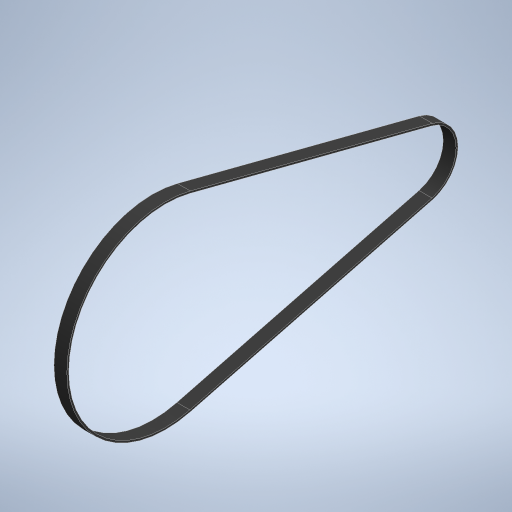
# Autodesk Inventor part: 射出_type1
Saved by Autodesk Inventor 2023 (Build 270158000, 158)
## iProperties
Created: 2022-04-20
Part Number: 射出_type1
Material: ゴム
Document SubType Name: Modeling
Designer: yuta
Density: 0.93 g/cm^3
Appearance: ゴム - 黒
Author: yuta
Autodesk Inventor part; units mm, degrees
ref_plane "YZ Plane" through (0, 0, 0) normal (1, 0, 0) x (0, 1, 0)
ref_plane "XZ Plane" through (0, 0, 0) normal (0, 1, 0) x (-1, 0, 0)
ref_plane "XY Plane" through (0, 0, 0) normal (0, 0, 1) x (1, 0, 0)
sketch "スケッチ1" plane through (0, 0, 0) normal (1, 0, 0) x (0, 1, 0)
  arc A0 (74.0708, -19.125) -> (-74.0708, -19.125) centre (0, 0) ccw
  arc A1 (-25.6585, -206.625) -> (25.6585, -206.625) centre (0, -200) ccw
  line L0 (74.0708, -19.125) -> (25.6585, -206.625)
  line L1 (-74.0708, -19.125) -> (-25.6585, -206.625)
  arc A2 (72.6184, -18.75) -> (-72.6184, -18.75) centre (0, 0) ccw
  arc A3 (-24.2061, -206.25) -> (24.2061, -206.25) centre (0, -200) ccw
  line L2 (-72.6184, -18.75) -> (-24.2061, -206.25)
  line L3 (72.6184, -18.75) -> (24.2061, -206.25)
  point P0 (26.5, -200)
  point P1 (-26.5, -200)
  point P2 (-26.5, -200)
  point P3 (25, -200)
  point P4 (-25, -200)
  point P5 (-62.2511, -58.9026)
  point P6 (-30.0666, -183.5524)
  dimension "d0" = 153
  dimension "d1" = 53
  dimension "d2" = 200
  dimension "d3" = 200
  dimension "d4" = 150
  dimension "d5" = 50
  dimension "d6" = 200
  constraints: 12 point on circle, 8 end point, 8 tangent, 4 centre point, 4 coincident, 2 point on line
  measures "d0" diameter of A0
  measures "d1" diameter of A1
  measures "d2" distance of point (0, 0) A1.centre
  measures "d3" vertical distance of point (0, 0) point (26.5, -200)
  measures "d4" diameter of A2
  measures "d5" diameter of A3
  measures "d6" vertical distance of point (0, 0) point (25, -200)
extrude "押し出し1" add sketch "スケッチ1" along normal blind 10
